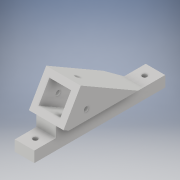
# Autodesk Inventor part: 30DegreeAttachementV02
Saved by Autodesk Inventor 2019.3 (Build 233278000, 278)
## iProperties
Created: 2019-02-16
Part Number: 30DegreeAttachementV02
Material: Generic
Document SubType Name: Modeling
Designer: steele
Density: 1 g/cm^3
Appearance: Default
Author: steele
Autodesk Inventor part; units mm, degrees
note: some values were not read from the file. Chosen so that the rebuilt part matches the saved one: direction of "Hole2".
ref_plane "YZ Plane" through (0, 0, 0) normal (1, 0, 0) x (0, 1, 0)
ref_plane "XZ Plane" through (0, 0, 0) normal (0, 1, 0) x (-1, 0, 0)
ref_plane "XY Plane" through (0, 0, 0) normal (0, 0, 1) x (1, 0, 0)
sketch "Sketch1" plane through (0, 0, 0) normal (1, 0, 0) x (0, 1, 0)
  line L0 (0, 0) -> (12.4509, 21.5656)
  line L1 (12.4509, 21.5656) -> (47.6462, 1.2456)
  line L2 (0, -101.8491) -> (0, 42.1347) projected
  line L3 (47.6462, 1.2456) -> (0, -81.28)
  line L4 (0, 0) -> (0, -81.28)
  line L5 (19.05, 17.7556) -> (0, -15.24) construction
  dimension "d0" = 40.64
  dimension "d1" = 30
  dimension "d5" = 7.62
  dimension "d6" = 38.1
  constraints: 10 end point, 3 point on line, 2 parallel, 1 collinear, 1 perpendicular
  measures "d0" distance of L0.end L1.end
  measures "d1" angle of L0 L2
  measures "d5" distance between parallel lines of L5 L0
  measures "d6" distance from line of L5.end L1
extrude "Extrusion1" add sketch "Sketch1" along normal mid plane 40.64
sketch "Sketch2" plane through (-20.32, 12.4509, 21.5656) normal (0, 0.5, 0.8660254) x (1, 0, 0)
  line L0 (0, 0) -> (40.64, 0) construction
  line L1 (40.64, 0) -> (40.64, 40.64) construction
  line L2 (0, 0) -> (40.64, 40.64) construction
  line L3 (40.64, 40.64) -> (0, 40.64) construction
  line L4 (0, 40.64) -> (40.64, 0) construction
  line L5 (7.62, 7.62) -> (33.02, 7.62)
  line L6 (33.02, 7.62) -> (33.02, 33.02)
  line L7 (33.02, 33.02) -> (7.62, 33.02)
  line L8 (7.62, 33.02) -> (7.62, 7.62)
  line L9 (7.62, 7.62) -> (33.02, 33.02) construction
  line L10 (33.02, 7.62) -> (7.62, 33.02) construction
  point P0 (20.32, 0)
  point P1 (20.32, 20.32)
  dimension "d7" = 25.4
  constraints: 16 end point, 3 midpoint, 2 parallel, 2 perpendicular, 1 horizontal
  measures "d7" distance of L7.end L5.start
extrude "Extrusion2" cut sketch "Sketch2" against normal blind 38.1
sketch "Sketch3" plane through (0, 0, 0) normal (1, 0, 0) x (0, 1, 0)
  line L0 (12.4509, 21.5656) -> (0, 0) projected
  line L1 (0, 0) -> (0, -81.28) projected
  line L2 (0, -81.28) -> (47.6462, 1.2456) projected
  line L3 (21.997, -27.94) -> (0, -15.24) projected
  line L4 (19.05, 17.7556) -> (0, -15.24) projected
  line L5 (0, 0) -> (0, -81.28)
  line L6 (12.4509, 21.5656) -> (-1.0999, 21.5656) construction
  line L7 (0, 0) -> (12.4509, 21.5656) projected
  line L8 (0, 0) -> (0, 46.9656)
  line L9 (47.6462, 1.2456) -> (0, -81.28) projected
  line L10 (0, -81.28) -> (0, -106.68)
  line L11 (0, -137.7901) -> (0, 79.9807) projected
  line L12 (0, 46.9656) -> (-12.7, 46.9656)
  line L13 (-12.7, 46.9656) -> (-12.7, -106.68)
  line L14 (-12.7, -106.68) -> (0, -106.68)
  point P0 (1.0999, -13.335)
  dimension "d10" = 25.4
  dimension "d11" = 25.4
  dimension "d12" = 12.7
  dimension "supportBaseLength" = 153.6456
  constraints: 14 end point, 5 vertical, 2 horizontal, 2 perpendicular, 2 other
  measures "d10" distance from line of L8.end L6
  measures "d11" distance of L1.end L10.end
  measures "d12" distance of L8.end L12.end
  measures "supportBaseLength" distance between parallel lines of L14 L12
extrude "Extrusion3" add sketch "Sketch3" along normal mid plane 22.86
sketch "Sketch5" plane through (0, 0, 0) normal (1, 0, 0) x (0, 1, 0)
  line L0 (0, 0) -> (12.4509, 21.5656) projected
  line L1 (0, 46.9656) -> (0, 0) projected
  line L2 (12.4509, 21.5656) -> (47.6462, 1.2456) projected
  line L3 (12.4509, 21.5656) -> (0, 21.5656)
  line L4 (0, 0) -> (12.4509, 21.5656)
  constraints: 4 end point, 1 horizontal, 1 point on line
extrude "Extrusion5" add sketch "Sketch5" along normal mid plane 22.86
sketch "Sketch4" plane through (0, 0, 0) normal (0, 0, 1) x (1, 0, 0)
  line L0 (20.32, 47.6462) -> (-20.32, 47.6462) projected
  line L1 (20.32, 0) -> (20.32, 47.6462) projected
  line L2 (20.32, 0) -> (11.43, 0) projected
  line L3 (11.43, 0) -> (-11.43, 0) projected
  line L4 (-11.43, 0) -> (-20.32, 0) projected
  line L5 (-20.32, 47.6462) -> (-20.32, 0) projected
  line L6 (-11.43, 0) -> (-11.43, -12.7) projected
  line L7 (11.43, -12.7) -> (-11.43, -12.7) projected
  line L8 (11.43, -12.7) -> (11.43, 0) projected
  line L9 (-11.43, 0) -> (-20.32, 8.89)
  line L10 (-20.32, 47.6462) -> (-20.32, 0) projected
  line L11 (-20.32, 8.89) -> (-20.32, 0)
  line L12 (0, 0) -> (0, 47.6462) construction
  line L13 (11.43, 0) -> (20.32, 0)
  line L14 (11.43, 0) -> (20.32, 8.89)
  line L15 (20.32, 8.89) -> (20.32, 0)
  dimension "d15" = 45
  constraints: 12 end point, 1 collinear, 1 midpoint, 1 point on line, 1 symmetric about line
  measures "d15" angle of L9 L4
extrude "Extrusion4" cut sketch "Sketch4" against normal up to surface (153.6456 mm away) from surface at 46.9656 contours L1 L2 L14 | L9 L4 L5
sketch "Sketch6" plane through (-11.43, 0, 46.9656) normal (0, 1, 0) x (1, 0, 0)
  line L0 (22.86, 153.6456) -> (0, 153.6456) construction
  line L1 (11.43, 153.6456) -> (11.43, 0) construction
  line L2 (22.86, 0) -> (0, 0) construction
  point P0 (11.43, 46.9656)
  point P1 (11.43, 140.9456)
  point P2 (11.43, 12.7)
  dimension "d21" = 12.7
  dimension "d22" = 12.7
  constraints: 2 end point, 2 midpoint, 2 point on line
  measures "d21" distance from line of point (11.43, 12.7) L2
  measures "d22" distance from line of point (11.43, 140.946) L0
hole "Hole1" at (0, 0, -93.98) at (0, 0, 34.2656) direction (0, -1, 0) diameter 5.6134 end through all clearance for "Flat Head Machine Screw (82)" size "#10" standard "Ansi Unified Screw Threads"
sketch "Sketch9" plane through (0, 0, 0) normal (1, 0, 0) x (0, 1, 0)
  line L0 (1.27, -13.0403) -> (1.27, -15.9732) projected
  line L1 (1.27, -15.9732) -> (21.997, -27.94) projected
  line L2 (41.047, 5.0556) -> (21.997, -27.94) projected
  line L3 (19.05, 17.7556) -> (41.047, 5.0556) projected
  line L4 (19.05, 17.7556) -> (1.27, -13.0403) projected
  line L5 (30.0485, 11.4056) -> (10.9985, -21.59) construction
  line L6 (1.27, -15.9732) -> (21.997, -27.94) construction
  circle A0 centre (20.5235, -5.0922) radius 2.8067
  point P0 (0, 0)
  dimension "d30" = 5.6134
  constraints: 2 end point, 2 midpoint, 1 centre point, 1 perpendicular, 1 point on line
  measures "d30" diameter of A0
extrude "Extrusion6" cut sketch "Sketch9" along normal through all both and the other way through all contours A0
sketch "Sketch10" plane through (-20.32, 47.6462, 1.2456) normal (0, 0.8660254, -0.5) x (1, 0, 0)
  line L0 (7.62, 0) -> (33.02, 0) construction
  line L1 (20.32, 0) -> (20.32, 77.7875) construction
  point P0 (20.32, 24.9018)
  point P1 (20.32, 19.05)
  dimension "d33" = 19.05
  constraints: 2 end point, 1 midpoint, 1 point on line, 1 vertical
  measures "d33" distance from line of point (20.32, 19.05) L0
hole "Hole2" at (0, 38.1212, -15.2522) direction (0, -0.8660254, 0.5) diameter 5.6134 depth 7.62 clearance for "Flat Head Machine Screw (82)" size "#10" standard "Ansi Unified Screw Threads"
equation "\"d0\" = widthToSupportExtrusion"
equation "\"d1\" = attachementAngle"
equation "\"d6\" = insertDepth"
equation "\"d2\" = widthToSupportExtrusion"
equation "\"d7\" = extrusionSize"
equation "\"d8\" = insertDepth"
equation "\"d12\" = supportBaseDepth"
equation "\"d13\" = supportBaseWidth"
equation "\"attachementAngle\" = 30deg"
equation "\"extrusionSize\" = 25.4"
equation "\"wallThickness\" = 6.35"
equation "\"slipClearance\" = 1.27"
equation "\"insertForExtrusion\" = extrusionSize + 2 * slipClearance"
equation "\"widthToSupportExtrusion\" = insertForExtrusion + 2 * wallThickness"
equation "\"insertDepth\" = 38.1"
equation "\"supportBaseWidth\" = 22.86"
equation "\"supportBaseDepth\" = 12.7"
body "Solid1"
